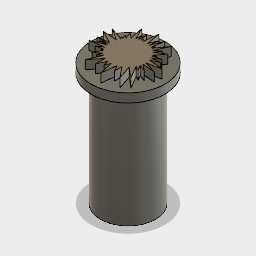
sunstamp (Autodesk Fusion 360 design; units mm, degrees)
Autodesk Fusion 360 part; units mm, degrees
cylinder "CylinderPrimitive1" add diameter 50 height 90 placed x (1, 0, 0) y (0, 0, -1) z (0, 1, 0) at (0, 0, 0) makes body 1
sketch "Sketch2" plane through (0, 90, 0) normal (0, 1, 0) x (-1, 0, 0)
  circle A0 centre (0, 0) radius 25
  circle A1 centre (0, 0) radius 29.446
extrude "Extrude1" add sketch "Sketch2" along normal blind 7 separate body makes body 2
sketch "Sketch3" plane through (0, 90, 0) normal (0, 1, 0) x (-1, 0, 0)
  circle A0 centre (0, 0) radius 25
extrude "Extrude2" add sketch "Sketch3" along normal blind 7 bodies 1 2
sketch "Sketch4" plane through (0, 97, 0) normal (0, 1, 0) x (-1, 0, 0)
  circle A0 centre (0, 0) radius 29.446
  circle A1 centre (0, 0) radius 14.1421
extrude "Extrude3" add sketch "Sketch4" along normal blind 5 contours A1 bodies 1
sketch "Sketch5" plane through (0, 97, 0) normal (0, 1, 0) x (-1, 0, 0)
  circle A0 centre (0, 0) radius 14.1421
  circle A1 centre (0, 0) radius 29.446
  line L0 (1.5459, -14.0574) -> (0.3849, -24.997)
  line L1 (0.3849, -24.997) -> (-1.6566, -14.0448)
  line L2 (-1.6566, -14.0448) -> (-4, -20)
  line L3 (-4, -20) -> (-3.5792, -13.6817)
  line L4 (-3.5792, -13.6817) -> (-6.9497, -22.2471)
  line L5 (-6.9497, -22.2471) -> (-5.5584, -13.004)
  line L6 (-5.5584, -13.004) -> (-6.9497, -14.718)
  line L7 (-6.9497, -14.718) -> (-6.6157, -12.4993)
  line L8 (-6.6157, -12.4993) -> (-13.0297, -21.3361)
  line L9 (-13.0297, -21.3361) -> (-8.5302, -11.2799)
  line L10 (-8.5302, -11.2799) -> (-12.9072, -14.718)
  line L11 (-12.9072, -14.718) -> (-9.9943, -10.0057)
  line L12 (-9.9943, -10.0057) -> (-16.9214, -14.718)
  line L13 (-16.9214, -14.718) -> (-11.6715, -7.986)
  line L14 (-11.6715, -7.986) -> (-14.2964, -8.6968)
  line L15 (-14.2964, -8.6968) -> (-12.242, -7.0805)
  line L16 (-12.242, -7.0805) -> (-18.2115, -8.6968)
  line L17 (-18.2115, -8.6968) -> (-13.0815, -5.3734)
  line L18 (-13.0815, -5.3734) -> (-20, -6)
  line L19 (-20, -6) -> (-13.7315, -3.3831)
  line L20 (-13.7315, -3.3831) -> (-24.912, -2.096)
  line L21 (-24.912, -2.096) -> (-14.1421, 0)
  line L22 (-14.1421, 0) -> (-24, 3)
  line L23 (-24, 3) -> (-13.9789, 2.1425)
  line L24 (-13.9789, 2.1425) -> (-18.9895, 6.0449)
  line L25 (-18.9895, 6.0449) -> (-13.5789, 3.9514)
  line L26 (-13.5789, 3.9514) -> (-16.2842, 8.2597)
  line L27 (-16.2842, 8.2597) -> (-12.6881, 6.2459)
  circle A2 centre (0, 0) radius 25
  line L28 (-12.6881, 6.2459) -> (-18.7739, 16.5089)
  line L29 (-18.7739, 16.5089) -> (-10.4839, 9.4915)
  line L30 (-10.4839, 9.4915) -> (-14.1957, 20.5787)
  line L31 (-14.1957, 20.5787) -> (-7.3108, 12.1059)
  line L32 (-7.3108, 12.1059) -> (-7.3108, 18)
  line L33 (-7.3108, 18) -> (-4.6794, 13.3455)
  line L34 (-4.6794, 13.3455) -> (-3.2491, 24.788)
  line L35 (-3.2491, 24.788) -> (-0.8759, 14.115)
  line L36 (-0.8759, 14.115) -> (1, 18)
  line L37 (1, 18) -> (1.8859, 14.0158)
  line L38 (1.8859, 14.0158) -> (5.1142, 20.702)
  line L39 (5.1142, 20.702) -> (5.1445, 13.1732)
  line L40 (5.1445, 13.1732) -> (12.046, 21.9065)
  line L41 (12.046, 21.9065) -> (7.7794, 11.8102)
  line L42 (7.7794, 11.8102) -> (10.9986, 14)
  line L43 (10.9986, 14) -> (9.4406, 10.5297)
  line L44 (9.4406, 10.5297) -> (14.5419, 13.9998)
  line L45 (14.5419, 13.9998) -> (11.2886, 8.5186)
  line L46 (11.2886, 8.5186) -> (12.8819, 8.5186)
  line L47 (12.8819, 8.5186) -> (12.1024, 7.3165)
  line L48 (12.1024, 7.3165) -> (17.5498, 8.5533)
  line L49 (17.5498, 8.5533) -> (13.0086, 5.5477)
  line L50 (13.0086, 5.5477) -> (23.9739, 7.0888)
  line L51 (23.9739, 7.0888) -> (13.7703, 3.2218)
  line L52 (13.7703, 3.2218) -> (19.4864, 3.2218)
  line L53 (19.4864, 3.2218) -> (13.9969, 2.0218)
  line L54 (13.9969, 2.0218) -> (23.2789, 1.3979)
  line L55 (23.2789, 1.3979) -> (14.1299, 0.5893)
  line L56 (14.1299, 0.5893) -> (24.5171, -4.8901)
  line L57 (24.5171, -4.8901) -> (13.5215, -4.1437)
  line L58 (13.5215, -4.1437) -> (22.7926, -10.2713)
  line L59 (22.7926, -10.2713) -> (12.4815, -6.6493)
  line L60 (12.4815, -6.6493) -> (13.3113, -8.5395)
  line L61 (13.3113, -8.5395) -> (11.8272, -7.7535)
  line L62 (11.8272, -7.7535) -> (13.2722, -11.0451)
  line L63 (13.2722, -11.0451) -> (10.8052, -9.124)
  line L64 (10.8052, -9.124) -> (12.5431, -14.3043)
  line L65 (12.5431, -14.3043) -> (8.7354, -11.1217)
  line L66 (8.7354, -11.1217) -> (11.0015, -22)
  line L67 (11.0015, -22) -> (6.4027, -12.7121)
  line L68 (6.4027, -12.7121) -> (6.4027, -17.0002)
  line L69 (6.4027, -17.0002) -> (4.7558, -13.3185)
  line L70 (4.7558, -19.3551) -> (3.323, -13.7462)
  line L71 (4.7558, -19.3551) -> (4.7558, -13.3185)
  line L72 (3.323, -13.7462) -> (2.6651, -15.1593)
  line L73 (2.6651, -15.1593) -> (1.5459, -14.0574)
  point P0 (-14.1421, 0)
sketch "Sketch6" plane through (0, 97, 0) normal (0, 1, 0) x (-1, 0, 0)
extrude "Extrude4" add sketch "Sketch5" along normal blind 5 contours A0 L56 L57 | A0 L54 L55 | A0 L58 L59 | A0 L52 L53 | A0 L60 L61 | A0 L50 L51 | A0 L62 L63 | A0 L0 L1 | A0 L48 L49 | A0 L64 L65 | A0 L72 L73 | A0 L2 L3 | A0 L8 L9 | A0 L46 L47 | A0 L40 L41 | A0 L66 L67 L68 L69 | A0 L70 L71 | A0 L4 L5 | A0 L6 L7 | A0 L10 L11 | A0 L20 L21 | A0 L44 L45 | A0 L34 L35 | A0 L38 L39 | A0 L42 L43 | A0 L12 L13 | A0 L18 L19 | A0 L22 L23 | A0 L28 L29 | A0 L30 L31 | A0 L32 L33 | A0 L36 L37 | A0 L14 L15 | A0 L16 L17 | A0 L24 L25 | A0 L26 L27 bodies 1
move_face "OffsetFaces1" offset -3 1 faces at (24.8758, 60, -2.4892) on bodies 1
move_face "OffsetFaces2" offset 2 1 faces at (0.2035, 102, 4.2512) on bodies 1
sketch "Sketch7" plane through (0, 104, 0) normal (0, 1, 0) x (-1, 0, 0)
  line L0 (-13.7315, -3.3831) -> (-20, -6)
  line L1 (-20, -6) -> (-13.0815, -5.3734)
  line L2 (-13.0815, -5.3734) -> (-18.2115, -8.6968)
  line L3 (-18.2115, -8.6968) -> (-12.242, -7.0805)
  line L4 (-12.242, -7.0805) -> (-14.2964, -8.6968)
  line L5 (-14.2964, -8.6968) -> (-11.6715, -7.986)
  line L6 (-11.6715, -7.986) -> (-16.9214, -14.718)
  line L7 (-16.9214, -14.718) -> (-9.9943, -10.0057)
  line L8 (-9.9943, -10.0057) -> (-12.9072, -14.718)
  line L9 (-12.9072, -14.718) -> (-8.5302, -11.2799)
  line L10 (-8.5302, -11.2799) -> (-13.0297, -21.3361)
  line L11 (-13.0297, -21.3361) -> (-6.6157, -12.4993)
  line L12 (-6.6157, -12.4993) -> (-6.9497, -14.718)
  line L13 (-6.9497, -14.718) -> (-5.5584, -13.004)
  line L14 (-5.5584, -13.004) -> (-6.9497, -22.2471)
  line L15 (-6.9497, -22.2471) -> (-3.5792, -13.6817)
  line L16 (-3.5792, -13.6817) -> (-4, -20)
  line L17 (-4, -20) -> (-1.6566, -14.0448)
  line L18 (-1.6566, -14.0448) -> (0.3849, -24.997)
  line L19 (0.3849, -24.997) -> (1.5459, -14.0574)
  line L20 (1.5459, -14.0574) -> (2.6651, -15.1593)
  line L21 (2.6651, -15.1593) -> (3.323, -13.7462)
  line L22 (3.323, -13.7462) -> (4.7558, -19.3551)
  line L23 (4.7558, -19.3551) -> (4.7558, -13.3185)
  line L24 (4.7558, -13.3185) -> (6.4027, -17.0002)
  line L25 (6.4027, -17.0002) -> (6.4027, -12.7121)
  line L26 (6.4027, -12.7121) -> (11.0015, -22)
  line L27 (11.0015, -22) -> (8.7354, -11.1217)
  line L28 (8.7354, -11.1217) -> (12.5431, -14.3043)
  line L29 (12.5431, -14.3043) -> (10.8052, -9.124)
  line L30 (10.8052, -9.124) -> (13.2722, -11.0451)
  line L31 (13.2722, -11.0451) -> (11.8272, -7.7535)
  line L32 (11.8272, -7.7535) -> (13.3113, -8.5395)
  line L33 (13.3113, -8.5395) -> (12.4815, -6.6493)
  line L34 (12.4815, -6.6493) -> (22.7926, -10.2713)
  line L35 (22.7926, -10.2713) -> (13.5215, -4.1437)
  line L36 (13.5215, -4.1437) -> (24.5171, -4.8901)
  line L37 (24.5171, -4.8901) -> (14.1299, 0.5893)
  line L38 (14.1299, 0.5893) -> (23.2789, 1.3979)
  line L39 (23.2789, 1.3979) -> (13.9969, 2.0218)
  line L40 (13.9969, 2.0218) -> (19.4864, 3.2218)
  line L41 (19.4864, 3.2218) -> (13.7703, 3.2218)
  line L42 (13.7703, 3.2218) -> (23.9739, 7.0888)
  line L43 (23.9739, 7.0888) -> (13.0086, 5.5477)
  line L44 (13.0086, 5.5477) -> (17.5498, 8.5533)
  line L45 (17.5498, 8.5533) -> (12.1024, 7.3165)
  line L46 (12.1024, 7.3165) -> (12.8819, 8.5186)
  line L47 (12.8819, 8.5186) -> (11.2886, 8.5186)
  line L48 (11.2886, 8.5186) -> (14.5419, 13.9998)
  line L49 (14.5419, 13.9998) -> (9.4406, 10.5297)
  line L50 (9.4406, 10.5297) -> (10.9986, 14)
  line L51 (10.9986, 14) -> (7.7794, 11.8102)
  line L52 (7.7794, 11.8102) -> (12.046, 21.9065)
  line L53 (12.046, 21.9065) -> (5.1445, 13.1732)
  line L54 (5.1445, 13.1732) -> (5.1142, 20.702)
  line L55 (5.1142, 20.702) -> (1.8859, 14.0158)
  line L56 (1.8859, 14.0158) -> (1, 18)
  line L57 (1, 18) -> (-0.8759, 14.115)
  line L58 (-0.8759, 14.115) -> (-3.2491, 24.788)
  line L59 (-3.2491, 24.788) -> (-4.6794, 13.3455)
  line L60 (-4.6794, 13.3455) -> (-7.3108, 18)
  line L61 (-7.3108, 18) -> (-7.3108, 12.1059)
  line L62 (-7.3108, 12.1059) -> (-14.1957, 20.5787)
  line L63 (-14.1957, 20.5787) -> (-10.4839, 9.4915)
  line L64 (-10.4839, 9.4915) -> (-18.7739, 16.5089)
  line L65 (-18.7739, 16.5089) -> (-12.6881, 6.2459)
  line L66 (-12.6881, 6.2459) -> (-16.2842, 8.2597)
  line L67 (-16.2842, 8.2597) -> (-13.5789, 3.9514)
  line L68 (-13.5789, 3.9514) -> (-18.9895, 6.0449)
  line L69 (-18.9895, 6.0449) -> (-13.9789, 2.1425)
  line L70 (-13.9789, 2.1425) -> (-24, 3)
  line L71 (-24, 3) -> (-14.1421, 0)
  line L72 (-14.1421, 0) -> (-24.912, -2.096)
  line L73 (-24.912, -2.096) -> (-13.7315, -3.3831)
